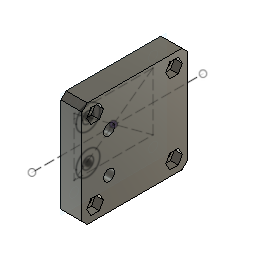
StagingPlateValveAdapter (Autodesk Fusion 360 design; units mm, degrees)
Autodesk Fusion 360 part; units mm, degrees
sketch "ValveAdapterBase" plane through (0, 0, 0) normal (1, 0, 0) x (0, 1, 0) in component "ValveHalterung"
  line L0 (-15, 15) -> (15, 15) construction
  line L1 (15, 15) -> (15, -15) construction
  line L2 (15, -15) -> (-15, -15) construction
  line L3 (-15, -15) -> (-15, 15) construction
  line L4 (-15, 15) -> (15, -15) construction
  line L5 (15, 15) -> (-15, -15) construction
  circle A0 centre (15, 15) radius 1.7
  circle A1 centre (15, -15) radius 1.7
  circle A2 centre (-15, -15) radius 1.7
  circle A3 centre (-15, 15) radius 1.7
  line L6 (-20, 20) -> (20, 20)
  line L7 (20, 20) -> (20, -20)
  line L8 (20, -20) -> (-20, -20)
  line L9 (-20, -20) -> (-20, 20)
  line L10 (-20, 20) -> (20, -20) construction
  line L11 (20, 20) -> (-20, -20) construction
  line L12 (-16.5877, 17.75) -> (-18.1754, 15)
  line L13 (-18.1754, 15) -> (-16.5877, 12.25)
  line L14 (-16.5877, 12.25) -> (-13.4123, 12.25)
  line L15 (-13.4123, 12.25) -> (-11.8246, 15)
  line L16 (-11.8246, 15) -> (-13.4123, 17.75)
  line L17 (-13.4123, 17.75) -> (-16.5877, 17.75)
  line L18 (0, 33) -> (0, -35) construction
  line L19 (41, 0) -> (-42, 0) construction
  line L20 (11.8246, 15) -> (13.4123, 17.75)
  line L21 (13.4123, 17.75) -> (16.5877, 17.75)
  line L22 (16.5877, 17.75) -> (18.1754, 15)
  line L23 (18.1754, 15) -> (16.5877, 12.25)
  line L24 (13.4123, 12.25) -> (11.8246, 15)
  line L25 (16.5877, 12.25) -> (13.4123, 12.25)
  line L26 (-18.1754, -15) -> (-16.5877, -12.25)
  line L27 (-16.5877, -12.25) -> (-13.4123, -12.25)
  line L28 (-13.4123, -12.25) -> (-11.8246, -15)
  line L29 (-11.8246, -15) -> (-13.4123, -17.75)
  line L30 (-16.5877, -17.75) -> (-18.1754, -15)
  line L31 (-13.4123, -17.75) -> (-16.5877, -17.75)
  line L32 (18.1754, -15) -> (16.5877, -12.25)
  line L33 (16.5877, -12.25) -> (13.4123, -12.25)
  line L34 (13.4123, -12.25) -> (11.8246, -15)
  line L35 (11.8246, -15) -> (13.4123, -17.75)
  line L36 (16.5877, -17.75) -> (18.1754, -15)
  line L37 (13.4123, -17.75) -> (16.5877, -17.75)
  circle A4 centre (7.3158, 9.4632) radius 2.1
  point P0 (-15, 15)
  dimension "d4" = 30
  dimension "d7" = 3.4
  dimension "d8" = 3.4
  dimension "d9" = 3.4
  dimension "d10" = 3.4
  dimension "d12" = 40
  dimension "d17" = 2.75
  dimension "d22" = 4.2
  constraint horizontal L0
  constraint perpendicular L0 L1
  constraint parallel L0 L2
  constraint parallel L1 L3
  constraint coincident L4 origin
  constraint coincident L5 origin
  constraint coincident L0.end L1.start
  constraint coincident L1.end L2.start
  constraint coincident L2.end L3.start
  constraint coincident P0 L0.start
  constraint horizontal L6
  constraint perpendicular L6 L7
  constraint parallel L6 L8
  constraint parallel L7 L9
  constraint coincident L10 origin
  constraint coincident L11 origin
  constraint equal L6 L7
  constraint equal L0 L1
  constraint horizontal L17
  constraint perpendicular L6 L18
  constraint horizontal L19
  constraint symmetric L12.start L18 L21.end
  constraint symmetric L12.end L18 L22.end
  constraint symmetric L13.end L18 L23.end
  constraint symmetric L14.end L18 L24.start
  constraint symmetric L15.end L18 L20.start
  constraint symmetric L16.end L18 L20.end
  constraint symmetric L12.start L19 L30.start
  constraint symmetric L12.end L19 L26.start
  constraint symmetric L13.end L19 L26.end
  constraint symmetric L14.end L19 L27.end
  constraint symmetric L15.end L19 L28.end
  constraint symmetric L16.end L19 L29.end
  constraint symmetric L19 L20.start L34.end
  constraint symmetric L19 L20.end L35.end
  constraint symmetric L19 L21.end L36.start
  constraint symmetric L19 L22.end L32.start
  constraint symmetric L19 L23.end L32.end
  constraint symmetric L19 L24.start L33.end
  measures "d4" distance of P0 L0.end
  measures "d7" diameter of A0
  measures "d8" diameter of A1
  measures "d9" diameter of A2
  measures "d10" diameter of A3
  measures "d12" distance of L6.start L6.end
  measures "d17" distance of P0 L17
  measures "d22" diameter of A4
extrude "Extrude1" add sketch "ValveAdapterBase" against normal blind 8 contours L6 L7 L8 L9 | L12 L13 L14 L15 L16 L17 | L20 L21 L22 L23 L24 L25 | L26 L27 L28 L29 L30 L31 | L32 L33 L34 L35 L36 L37 | A4 in component "ValveHalterung"
extrude "Extrude2" cut sketch "ValveAdapterBase" against normal blind 3 contours L12 L13 L14 L15 L16 L17 | L20 L21 L22 L23 L24 L25 | L26 L27 L28 L29 L30 L31 | L32 L33 L34 L35 L36 L37 in component "ValveHalterung"
sketch "ValveAdapterScrews" plane through (-8, 0, 0) normal (-1, 0, 0) x (0, -1, 0) in component "ValveHalterung"
  circle A0 centre (-15, 15) radius 1.7
  circle A1 centre (15, 15) radius 1.7
  circle A2 centre (-15, -15) radius 1.7
  circle A3 centre (15, -15) radius 1.7
  line L0 (-20, -20) -> (20, -20)
  line L1 (20, -20) -> (20, 20)
  line L2 (20, 20) -> (-20, 20)
  line L3 (-20, 20) -> (-20, -20)
  line L4 (-15, 11) -> (15, 11) construction
  line L5 (15, 11) -> (15, -11) construction
  line L6 (15, -11) -> (-15, -11) construction
  line L7 (-15, -11) -> (-15, 11) construction
  line L8 (-15, 11) -> (15, -11) construction
  line L9 (15, 11) -> (-15, -11) construction
  circle A4 centre (9.7, 7.1) radius 2.1
  line L10 (11.8, 7.1) -> (11.8, 11) construction
  line L11 (9.7, 9.2) -> (15, 9.2) construction
  line L12 (31, -0.4) -> (-34, -0.4) construction
  circle A5 centre (9.7, -7.9) radius 2.1
  circle A6 centre (9.7, 7.1) radius 4.5
  circle A7 centre (9.7, -7.9) radius 4.5
  dimension "d35" = 30
  dimension "d36" = 22
  dimension "d37" = 4.2
  dimension "d38" = 3.2
  dimension "d39" = 1.8
  dimension "d42" = 9
  dimension "d47" = 15
  constraint horizontal L4
  constraint perpendicular L4 L5
  constraint parallel L4 L6
  constraint parallel L5 L7
  constraint coincident L8 origin
  constraint coincident L9 origin
  constraint coincident A4 L10.start
  constraint coincident L4 L10.end
  constraint perpendicular L4 L10
  constraint tangent A4 L10
  constraint coincident A4 L11.start
  constraint coincident L5 L11.end
  constraint perpendicular L5 L11
  constraint tangent A4 L11
  constraint perpendicular L1 L12
  constraint symmetric A4 L12 A5
  constraint concentric A4 A6
  constraint symmetric L12 A6 A7
  measures "d35" distance of L5.end L6.end
  measures "d36" distance of L4.end L5.end
  measures "d37" diameter of A4
  measures "d38" distance of L5 L10
  measures "d39" distance of L4 L11
  measures "d42" diameter of A6
  measures "d47" distance of A5.centre A4.centre
extrude "Extrude3" cut sketch "ValveAdapterScrews" against normal up to surface (8 mm away) contours A4 | A5 in component "ValveHalterung"
extrude "Extrude4" cut sketch "ValveAdapterScrews" against normal blind 4.5 contours A6 | A7 in component "ValveHalterung"
chamfer "Chamfer1" distance 2 angle 45 4 edges at (-4, -20, 20) (-4, 20, 20) (-4, -20, -20) (-4, 20, -20) in component "ValveHalterung"
component "ValveHalterung" placed x (1, 0, 0) y (0, 1, 0) z (0, 0, 1) at (0, 0, 0)
equation "Staging_Plate_Spacing = 30 mm" comment "M3 Screws"
equation "d4 = Staging_Plate_Spacing"
equation "M3_Screw_Diameter = 3.4 mm"
equation "d7 = M3_Screw_Diameter"
equation "d8 = M3_Screw_Diameter"
equation "d9 = M3_Screw_Diameter"
equation "d10 = M3_Screw_Diameter"
equation "Outer_Edge = 40 mm"
equation "d12 = Outer_Edge"
equation "M3_Nut_Edge = 5.5 mm"
equation "d17 = M3_Nut_Edge / 2"
equation "M3_Nut_Extrusion = 3 mm"
equation "d19 = -M3_Nut_Extrusion"
equation "Valve_Screw_Diameter = 4.2 mm" comment "M4 Screw?"
equation "d22 = Valve_Screw_Diameter"
equation "d37 = Valve_Screw_Diameter"
equation "d42 = Valve_Screw_Head_Diameter"
equation "Valve_Screw_Head_Diameter = 9 mm"
